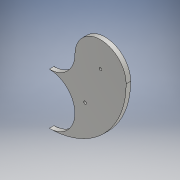
# Autodesk Inventor part: A0004
Saved by Autodesk Inventor 2017 (Build 210142000, 142)
## iProperties
Part Number: A0004
Material: 一般
Document SubType Name: Modeling
Designer: lygfy
Density: 1 g/cm^3
Appearance: 銅 - 緞
Author: lygfy
Autodesk Inventor part; units mm, degrees
ref_plane "YZ Plane" through (0, 0, 0) normal (1, 0, 0) x (0, 1, 0)
ref_plane "XZ Plane" through (0, 0, 0) normal (0, 1, 0) x (-1, 0, 0)
ref_plane "XY Plane" through (0, 0, 0) normal (0, 0, 1) x (1, 0, 0)
sketch "草圖1" plane through (0, 0, 0) normal (0, 1, 0) x (-1, 0, 0)
  arc A0 (-45, 0) -> (0, -45) centre (0, 0) ccw construction
  arc A1 (-67.5, 0) -> (0, -67.5) centre (0, 0) ccw
  arc A2 (-22.5, 0) -> (0, -22.5) centre (0, 0) ccw
  arc A3 (-22.5, 0) -> (-67.5, 0) centre (-45, 0) ccw
  arc A4 (0, -22.5) -> (0, -67.5) centre (0, -45) ccw
  dimension "d1" = 45
  dimension "d3" = 22.5
  constraints: 10 point on circle, 5 centre point, 2 coincident, 2 tangent, 1 equal radius, 1 horizontal alignment, 1 vertical alignment
  measures "d1" radius of A0
  measures "d3" radius of A3
extrude "擠出1" add sketch "草圖1" along normal blind 4
sketch "草圖3" plane through (0, 0, 0) normal (0, -1, 0) x (1, 0, 0)
  arc A0 (0, -45) -> (45, 0) centre (0, 0) ccw construction
  line L0 (45, 0) -> (31.3889, -32.245)
  dimension "d7" = 35
  constraints: 2 end point, 1 point on circle
  measures "d7" distance of L0.start L0.end
hole "孔1" at (45, 0, 0) at (31.3889, 0, -32.245) direction (0, 1, 0) diameter 2.459 end through all thread size "M3x0.5" class "6H" standard "ISO Metric profile"
